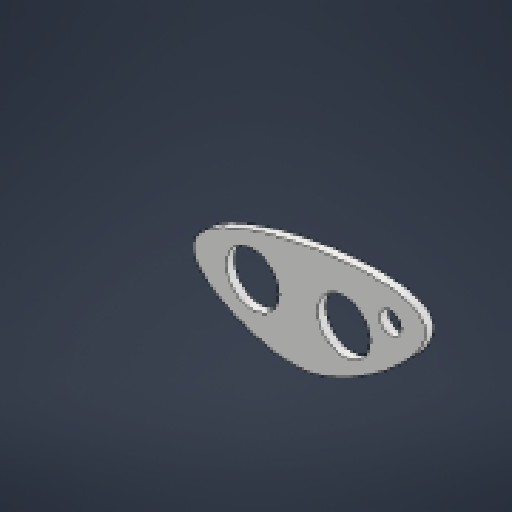
# Autodesk Inventor part: Endgame release polycarb
Saved by Autodesk Inventor 2023.2 (Build 272271030, 271C)
## iProperties
Created: 2023-05-29
Part Number: Endgame release polycarb
Material: Generic
Document SubType Name: Modeling
Designer: Main Account
Density: 1 g/cm^3
Appearance: Default
Author: Main Account
Autodesk Inventor part; units mm, degrees
ref_plane "YZ Plane" through (0, 0, 0) normal (1, 0, 0) x (0, 1, 0)
ref_plane "XZ Plane" through (0, 0, 0) normal (0, 1, 0) x (-1, 0, 0)
ref_plane "XY Plane" through (0, 0, 0) normal (0, 0, 1) x (1, 0, 0)
sketch "Sketch1" plane through (0, 0, 0) normal (0, 0, 1) x (1, 0, 0)
  circle A0 centre (-3.937, -6.8191) radius 1.7525 construction
  circle A1 centre (-3.937, -6.8191) radius 2.0986
  ellipse E0 centre (-12.9574, -11.8563) end of major axis (-9.9221, -11.8563) minor radius 3.01 construction
  ellipse E1 centre (-30.5618, -12.8333) end of major axis (-27.5265, -12.8333) minor radius 3.01 construction
  circle A2 centre (-12.9574, -11.8563) radius 5.08
  circle A3 centre (-30.5618, -12.8333) radius 5.08
  spline S0 degree 5 poles (-7.8774, -17.4136) (-2.4104, -13.5962) (6.4561, -5.325) (12.7977, 6.5892) (-74.198, -8.1833) (-29.9103, -23.3221) (-22.0988, -25.3968) (-13.1226, -21.076) (-7.8774, -17.4136) knots 0 0 0 0 0 0 0.306213 0.506213 0.706213 1 1 1 1 1 1
  point P0 (0, 0)
  point P1 (-41.7028, -11.8563)
  point P2 (-28.7309, -22.3933)
  dimension "d0" = 4.1971
  dimension "d1" = 10.16
  dimension "d2" = 10.16
  constraints: 3 centre point, 3 coincident, 8 other
  measures "d0" diameter of A1
  measures "d1" diameter of A2
  measures "d2" diameter of A3
extrude "Extrusion1" add sketch "Sketch1" along normal blind 1.5875
body "Solid1"
